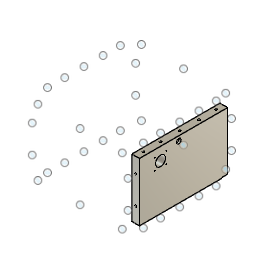
CAD_File 5 (Autodesk Fusion 360 design; units mm, degrees)
Autodesk Fusion 360 part; units mm, degrees
sketch "Sketch1" plane through (0, 0, -20) normal (0, 0, -1) x (1, 0, 0)
  circle A0 centre (15, 75) radius 1.5
  circle A1 centre (-15, 75) radius 1.5
  circle A2 centre (15, 45) radius 1.5
  circle A3 centre (-15, 45) radius 1.5
  circle A4 centre (0, 60) radius 14
  line L0 (-135, -115) -> (135, -115)
  line L1 (135, -115) -> (135, 115)
  line L2 (135, 115) -> (-135, 115)
  line L3 (-135, 115) -> (-135, -115)
  line L4 (135, 115) -> (115, 115)
  line L5 (115, 115) -> (115, -115)
  line L6 (115, -115) -> (135, -115)
  line L7 (135, -115) -> (135, 115)
  dimension "d484" = 20
  constraint horizontal L4
  constraint vertical L5
  constraint horizontal L6
  constraint vertical L7
  constraint coincident L1.end L2.start
  measures "d484" distance of L1.end L4.end
extrude "Extrude1" add sketch "Sketch1" along normal blind 152.35 contours L0 L1 L2 L4 L5 L6 L7
sketch "Sketch2" plane through (135, 0, 0) normal (1, 0, 0) x (0, 1, 0)
  line L0 (115, -20) -> (-115, -20)
  line L1 (-115, -20) -> (-115, -172.35)
  line L2 (-115, -172.35) -> (115, -172.35)
  line L3 (115, -172.35) -> (115, -20)
  circle A0 centre (-60, -53.02) radius 13
  circle A1 centre (-45, -38.02) radius 1.4224
  circle A2 centre (-45, -68.02) radius 1.4224
  circle A3 centre (-75, -68.02) radius 1.4224
  circle A4 centre (-75, -38.02) radius 1.4224
  dimension "d519" = 26
  measures "d519" diameter of A0
extrude "Extrude2" cut sketch "Sketch2" against normal up to surface (20 mm away) contours A0 | A1 | A2 | A3 | A4
thread "Thread1" "ANSI Unified Screw Threads 0.112(#4) 4-40 UNC 3B" major diameter 2.8448 minor diameter 2.2708 pitch 0.635 angle 60 resizes the face on face at (121.6667, -43.8662, -37.1611) on face at (121.6667, -43.5794, -68.0909) on face at (121.6667, -76.2137, -68.7617) on face at (121.6667, -75.247, -36.6192)
sketch "sketch 1965" plane through (0, 0, 0) normal (0, 0, 1) x (-1, 0, 0)
  circle A0 centre (-125, 0) radius 3
  circle A1 centre (125, 95) radius 3
  circle A2 centre (125, -95) radius 3
  circle A3 centre (125, 0) radius 3
  circle A4 centre (-125, 95) radius 3
  circle A5 centre (-125, -95) radius 3
extrude "Extrude3" cut sketch "sketch 1965" against normal blind 40
sketch "sketch 1998" plane through (0, 0, 0) normal (0, 0, 1) x (-1, 0, 0)
  circle A0 centre (-125, 50) radius 3
  circle A1 centre (125, -50) radius 3
  circle A2 centre (125, 50) radius 3
  circle A3 centre (-125, -50) radius 3
extrude "Extrude4" cut sketch "sketch 1998" against normal blind 35
sketch "sketch 2022" plane through (0, 0, -192.35) normal (0, 0, -1) x (1, 0, 0)
  circle A0 centre (125, 0) radius 3
  circle A1 centre (-125, 95) radius 3
  circle A2 centre (-125, -95) radius 3
  circle A3 centre (-125, 0) radius 3
  circle A4 centre (125, 95) radius 3
  circle A5 centre (125, -95) radius 3
extrude "Extrude5" cut sketch "sketch 2022" against normal blind 40
sketch "sketch 2054" plane through (0, 0, -192.35) normal (0, 0, -1) x (1, 0, 0)
  circle A0 centre (-125, -50) radius 3
  circle A1 centre (125, -50) radius 3
  circle A2 centre (125, 50) radius 3
  circle A3 centre (-125, 50) radius 3
extrude "Extrude6" cut sketch "sketch 2054" against normal blind 35
sketch "sketch 2078" plane through (0, 135, 0) normal (0, 1, 0) x (-1, 0, 0)
  circle A0 centre (-110, -182.35) radius 3
  circle A1 centre (110, -182.35) radius 3
  circle A2 centre (125, -60) radius 3
  circle A3 centre (0, -10) radius 3
  circle A4 centre (-125, -60) radius 3
  circle A5 centre (-110, -10) radius 3
  circle A6 centre (110, -10) radius 3
  circle A7 centre (125, -132.35) radius 3
  circle A8 centre (0, -182.35) radius 3
  circle A9 centre (-125, -132.35) radius 3
extrude "Extrude7" cut sketch "sketch 2078" against normal blind 40
sketch "sketch 2126" plane through (0, -135, 0) normal (0, -1, 0) x (1, 0, 0)
  circle A0 centre (-110, -182.35) radius 3
  circle A1 centre (110, -182.35) radius 3
  circle A2 centre (125, -60) radius 3
  circle A3 centre (0, -10) radius 3
  circle A4 centre (-125, -60) radius 3
  circle A5 centre (-110, -10) radius 3
  circle A6 centre (110, -10) radius 3
  circle A7 centre (125, -132.35) radius 3
  circle A8 centre (0, -182.35) radius 3
  circle A9 centre (-125, -132.35) radius 3
extrude "Extrude8" cut sketch "sketch 2126" against normal blind 40
thread "Thread2" "ISO Metric profile 6.0 M6x1 6H" major diameter 6.147 minor diameter 5.035 pitch 1 angle 60 resizes the face on face at (126.9851, 101.6667, -62.2493) on face at (127.6347, 93.5652, -165.6833) on face at (127.0947, -108.3333, -130.2024) on face at (123.7661, -2.7345, -165.6833) on face at (127.6347, -96.4348, -165.6833) on face at (122.3653, -96.4348, -26.6667) on face at (122.9053, 108.3333, -130.2024) on face at (123.0149, -101.6667, -62.2493) on face at (122.3653, 93.5652, -26.6667) on face at (126.2339, -2.7345, -26.6667)
sketch "Sketch3" plane through (0, 0, -172.35) normal (0, 0, -1) x (1, 0, 0)
  circle A0 centre (125, 50) radius 3
  circle A1 centre (125, -50) radius 3
  circle A2 centre (125, 95) radius 2.5175
  circle A3 centre (125, 0) radius 2.5175
  circle A4 centre (125, -95) radius 2.5175
  line L0 (135, -115) -> (135, 115)
  line L1 (135, 115) -> (115, 115)
  line L2 (115, 115) -> (115, -115)
  line L3 (115, -115) -> (135, -115)
  line L4 (115, -115) -> (135, -115)
  line L5 (135, -115) -> (135, -101)
  line L6 (135, -101) -> (115, -101)
  line L7 (115, -101) -> (115, -115)
  constraint horizontal L4
  constraint vertical L5
  constraint horizontal L6
  constraint vertical L7
  constraint coincident L0 L5.end
  constraint coincident L2.end L3.start
extrude "Extrude9" cut sketch "Sketch3" against normal blind 2 contours L0 L2 L3 L4 L5 L6 L7
sketch "Sketch5" plane through (115, 0, 0) normal (-1, 0, 0) x (0, -1, 0)
  line L0 (-115, -170.35) -> (-101, -170.35)
  line L1 (-101, -170.35) -> (-101, -172.35)
  line L2 (-101, -172.35) -> (115, -172.35)
  line L3 (115, -172.35) -> (115, -20)
  line L4 (115, -20) -> (-115, -20)
  line L5 (-115, -20) -> (-115, -170.35)
  circle A0 centre (45, -68.02) radius 1.1354
  circle A1 centre (60, -53.02) radius 13
  circle A2 centre (75, -68.02) radius 1.1354
  circle A3 centre (75, -38.02) radius 1.1354
  circle A4 centre (45, -38.02) radius 1.1354
  line L6 (82.3611, -147.4331) -> (83.589, -147.2693)
  spline S0 degree 2 poles (83.589, -147.2693) (83.8004, -148.313) (84.3086, -148.7734) knots 0 0 0 1 1 1
  spline S1 degree 2 poles (84.3086, -148.7734) (84.8168, -149.2339) (85.5467, -149.2339) knots 0 0 0 1 1 1
  spline S2 degree 2 poles (85.5467, -149.2339) (86.413, -149.2339) (87.0098, -148.6336) knots 0 0 0 1 1 1
  spline S3 degree 2 poles (87.0098, -148.6336) (87.6067, -148.0333) (87.6067, -147.1466) knots 0 0 0 1 1 1
  spline S4 degree 2 poles (87.6067, -147.1466) (87.6067, -146.3007) (87.0542, -145.7516) knots 0 0 0 1 1 1
  spline S5 degree 2 poles (87.0542, -145.7516) (86.5017, -145.2025) (85.649, -145.2025) knots 0 0 0 1 1 1
  spline S6 degree 2 poles (85.649, -145.2025) (85.3011, -145.2025) (84.7827, -145.3389) knots 0 0 0 1 1 1
  line L7 (84.7827, -145.3389) -> (84.9191, -144.2612)
  spline S7 degree 2 poles (84.9191, -144.2612) (85.0419, -144.2748) (85.1169, -144.2748) knots 0 0 0 1 1 1
  spline S8 degree 2 poles (85.1169, -144.2748) (85.9014, -144.2748) (86.5289, -143.8655) knots 0 0 0 1 1 1
  spline S9 degree 2 poles (86.5289, -143.8655) (87.1565, -143.4563) (87.1565, -142.6036) knots 0 0 0 1 1 1
  spline S10 degree 2 poles (87.1565, -142.6036) (87.1565, -141.9283) (86.6995, -141.4849) knots 0 0 0 1 1 1
  spline S11 degree 2 poles (86.6995, -141.4849) (86.2424, -141.0415) (85.5194, -141.0415) knots 0 0 0 1 1 1
  spline S12 degree 2 poles (85.5194, -141.0415) (84.8032, -141.0415) (84.3257, -141.4917) knots 0 0 0 1 1 1
  spline S13 degree 2 poles (84.3257, -141.4917) (83.8482, -141.9419) (83.7117, -142.8423) knots 0 0 0 1 1 1
  line L8 (83.7117, -142.8423) -> (82.4839, -142.6241)
  spline S14 degree 2 poles (82.4839, -142.6241) (82.709, -141.3894) (83.5071, -140.7107) knots 0 0 0 1 1 1
  spline S15 degree 2 poles (83.5071, -140.7107) (84.3052, -140.032) (85.4921, -140.032) knots 0 0 0 1 1 1
  spline S16 degree 2 poles (85.4921, -140.032) (86.3107, -140.032) (86.9996, -140.3833) knots 0 0 0 1 1 1
  spline S17 degree 2 poles (86.9996, -140.3833) (87.6886, -140.7346) (88.0535, -141.3417) knots 0 0 0 1 1 1
  spline S18 degree 2 poles (88.0535, -141.3417) (88.4184, -141.9488) (88.4184, -142.6309) knots 0 0 0 1 1 1
  spline S19 degree 2 poles (88.4184, -142.6309) (88.4184, -143.2789) (88.0705, -143.811) knots 0 0 0 1 1 1
  spline S20 degree 2 poles (88.0705, -143.811) (87.7227, -144.343) (87.0405, -144.6568) knots 0 0 0 1 1 1
  spline S21 degree 2 poles (87.0405, -144.6568) (87.9273, -144.8614) (88.4184, -145.506) knots 0 0 0 1 1 1
  spline S22 degree 2 poles (88.4184, -145.506) (88.9096, -146.1507) (88.9096, -147.1193) knots 0 0 0 1 1 1
  spline S23 degree 2 poles (88.9096, -147.1193) (88.9096, -148.429) (87.9546, -149.3396) knots 0 0 0 1 1 1
  spline S24 degree 2 poles (87.9546, -149.3396) (86.9996, -150.2503) (85.5398, -150.2503) knots 0 0 0 1 1 1
  spline S25 degree 2 poles (85.5398, -150.2503) (84.2233, -150.2503) (83.3536, -149.4658) knots 0 0 0 1 1 1
  spline S26 degree 2 poles (83.3536, -149.4658) (82.4839, -148.6814) (82.3611, -147.4331) knots 0 0 0 1 1 1
extrude "Extrude11" cut sketch "Sketch5" against normal blind 0.2 contours L6 S0 S1 S2 S3 S4 S5 S6 L7 S7 S8 S9 S10 S11 S12 S13 L8 S14 S15 S16 S17 S18 S19 S20 S21 S22 S23 S24 S25 S26
sketch "Sketch6" plane through (135, 0, 0) normal (1, 0, 0) x (0, 1, 0)
  line L0 (101, -170.35) -> (115, -170.35)
  line L1 (115, -170.35) -> (115, -20)
  line L2 (115, -20) -> (-115, -20)
  line L3 (-115, -20) -> (-115, -172.35)
  line L4 (-115, -172.35) -> (101, -172.35)
  line L5 (101, -172.35) -> (101, -170.35)
  circle A0 centre (-45, -38.02) radius 1.1354
  circle A1 centre (-75, -38.02) radius 1.1354
  circle A2 centre (-75, -68.02) radius 1.1354
  circle A3 centre (-60, -53.02) radius 13
  circle A4 centre (-45, -68.02) radius 1.1354
  circle A5 centre (-12.5, -32) radius 6
  dimension "d962" = 12
  dimension "d963" = 12
  dimension "d964" = 102.5
  measures "d962" diameter of A5
  measures "d963" distance of L2 A5.centre
  measures "d964" distance of L3 A5.centre
extrude "Extrude12" cut sketch "Sketch6" against normal blind 5 contours A5
